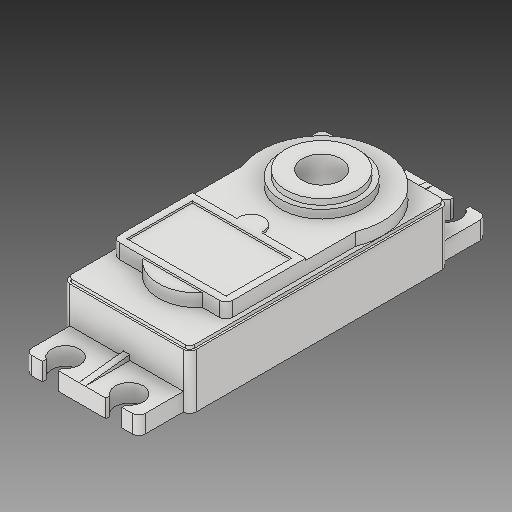
# Autodesk Inventor part: Top
Saved by Autodesk Inventor 2018 (Build 220112000, 112)
## iProperties
Created: 2016-09-26
Part Number: Top
Material: Plástico ABS
Document SubType Name: Modeling
Designer: Julian
Density: 1.06 g/cm^3
Appearance: Suave - Blanco
Author: Julian
Autodesk Inventor part; units mm, degrees
ref_plane "YZ Plane" through (0, 0, 0) normal (1, 0, 0) x (0, 1, 0)
ref_plane "XZ Plane" through (0, 0, 0) normal (0, 1, 0) x (-1, 0, 0)
ref_plane "XY Plane" through (0, 0, 0) normal (0, 0, 1) x (1, 0, 0)
sketch "Boceto1" plane through (0, 0, 0) normal (0, 1, 0) x (-1, 0, 0)
  line L0 (9.9, 20.3) -> (-9.9, 20.3)
  line L1 (-9.9, 20.3) -> (-9.9, -20.3)
  line L2 (-9.9, -20.3) -> (9.9, -20.3)
  line L3 (9.9, -20.3) -> (9.9, 20.3)
  line L4 (9.9, 20.3) -> (-9.9, -20.3) construction
  line L5 (-9.9, 20.3) -> (9.9, -20.3) construction
  point P0 (0, 0)
  dimension "d0" = 19.8
  dimension "d1" = 40.6
  constraints: 12 end point, 2 midpoint, 2 parallel, 1 horizontal, 1 perpendicular
  measures "d0" distance of L2.end L1.end
  measures "d1" distance of L1.end L0.end
extrude "Extrusión1" add sketch "Boceto1" against normal blind 9
sketch "Boceto2" plane through (0, 0, 0) normal (0, 1, 0) x (1, 0, 0)
  circle A0 centre (0, 10.3) radius 3
  line L0 (9.9, 20.3) -> (-9.9, 20.3) projected
  point P0 (0, 0)
  dimension "d4" = 6
  dimension "d5" = 10
  constraints: 1 centre point
  measures "d4" diameter of A0
  measures "d5" distance from line of L0 A0.centre
extrude "Extrusión2" cut sketch "Boceto2" against normal through all
sketch "Boceto5" plane through (0, -9, 0) normal (0, -1, 0) x (1, 0, 0)
  line L0 (-8.9, 20.3) -> (8.9, 20.3)
  line L1 (8.9, 20.3) -> (8.9, 27.3)
  line L2 (8.9, 27.3) -> (-8.9, 27.3)
  line L3 (-8.9, 27.3) -> (-8.9, 20.3)
  line L4 (-8.9, 20.3) -> (8.9, 27.3) construction
  line L5 (8.9, 20.3) -> (-8.9, 27.3) construction
  line L6 (-9.9, 27.3) -> (9.9, 27.3)
  line L7 (9.9, 20.3) -> (-9.9, 20.3) projected
  point P0 (0, 0)
  point P1 (0, 0)
  point P2 (0, 23.8)
  dimension "d23" = 17.8
  dimension "d24" = 7
  constraints: 14 end point, 2 collinear, 2 midpoint, 2 parallel, 1 horizontal, 1 perpendicular
  measures "d23" distance of L2.end L1.end
  measures "d24" distance of L1.end L0.end
extrude "Extrusión5" add sketch "Boceto5" against normal blind 2.8
sketch "Boceto6" plane through (0, -6.2, 0) normal (0, 1, 0) x (1, 0, 0)
  arc A0 (-3.75, -26.7004) -> (-6.25, -26.7004) centre (-5, -24.89) ccw
  line L0 (-8.9, -27.3) -> (8.9, -27.3)
  line L1 (-3.75, -27.3) -> (-6.25, -27.3)
  line L2 (-6.25, -27.3) -> (-6.25, -26.7)
  line L3 (-3.75, -26.7) -> (-3.75, -27.3)
  line L4 (0, -27.3) -> (0, -23.9124)
  line L5 (-8.9, -20.3) -> (-8.9, -27.3)
  line L6 (-8.9, -20.3) -> (8.9, -20.3) projected
  line L7 (-8.3229, -20.3) -> (8.9, -20.3)
  line L8 (8.9, -20.3) -> (8.9, -27.3)
  point P0 (0, 0)
  point P1 (0, 0)
  dimension "d27" = 4.4
  dimension "d28" = 2.41
  dimension "d29" = 5
  dimension "d30" = 2.65
  dimension "d31" = 0.6
  constraints: 16 end point, 3 point on line, 2 horizontal, 2 parallel, 2 perpendicular, 2 point on circle, 2 vertical, 1 centre point, 1 midpoint
  measures "d27" diameter of A0
  measures "d28" distance from line of L0 A0.centre
  measures "d29" distance from line of L4 A0.centre
  measures "d30" distance between parallel lines of L5 L2
  measures "d31" distance of L3.start L1.start
extrude "Extrusión6" cut sketch "Boceto6" against normal through all contours L3 L0 L2 A0
sketch "Boceto8" plane through (0, 0, 0) normal (1, 0, 0) x (0, 1, 0)
  line L0 (-6.2, 27.3) -> (-5.4, 20.3)
  line L1 (-5.4, 20.3) -> (-6.2, 20.3)
  line L2 (-6.2, 20.3) -> (-6.2, 27.3)
  point P0 (0, 0)
  dimension "d34" = 0.8
  constraints: 6 end point, 1 horizontal, 1 perpendicular
  measures "d34" distance of L1.end L0.end
extrude "Extrusión7" add sketch "Boceto8" along normal mid plane 1
mirror "Simetría3" about plane through (0, 0, 0) normal (1, 0, 0) of "Extrusión6"
mirror "Simetría4" about plane through (0, 0, 0) normal (0, 0, 1) of "Extrusión5", "Extrusión6", "Simetría3", "Extrusión7"
sketch "Boceto9" plane through (0, 0, 0) normal (0, 1, 0) x (1, 0, 0)
  circle A0 centre (0, 10.3) radius 3 projected
  line L0 (-8.9, -13.5986) -> (8.9, -13.5986)
  line L1 (8.9, -13.5986) -> (8.9, 6.7014)
  line L2 (-8.9, 6.7014) -> (-8.9, -13.5986)
  line L3 (-8.9, -13.5986) -> (5.885, 8.9919) construction
  line L4 (8.9, -13.5986) -> (-5.885, 8.9919) construction
  arc A1 (8.9, 6.7014) -> (-8.9, 6.7014) centre (0, 10.3) ccw
  line L5 (9.9, 20.3) -> (-9.9, 20.3) projected
  point P0 (0, 0)
  dimension "d40" = 9.6
  dimension "d42" = 20.3
  dimension "d61" = 17.8
  constraints: 10 end point, 2 parallel, 2 point on circle, 2 point on line, 1 centre point, 1 horizontal, 1 perpendicular
  measures "d40" radius of A1
  measures "d42" distance of L0.end L1.end
  measures "d61" distance between parallel lines of L1 L2
extrude "Extrusión8" add sketch "Boceto9" along normal blind 2
sketch "Boceto11" plane through (0, 2, 0) normal (0, 1, 0) x (1, 0, 0)
  line L0 (-8.9, -13.5986) -> (8.9, -13.5986) projected
  line L1 (5.2244, -15.7986) -> (5.2244, -13.5986)
  arc A0 (-4.1756, -13.5986) -> (5.2244, -13.5986) centre (0.5244, -9.6782) ccw
  line L2 (-4.1756, -13.5986) -> (5.2244, -13.5986)
  point P0 (0, 0)
  dimension "d50" = 2.2
  dimension "d51" = 9.4
  constraints: 4 end point, 2 point on circle, 1 centre point, 1 collinear, 1 point on line
  measures "d50" distance edge to line of A0 L0
  measures "d51" distance of L1.end L2.start
extrude "Extrusión9" add sketch "Boceto11" against normal blind 2
sketch "Boceto12" plane through (0, 2, 0) normal (0, 1, 0) x (1, 0, 0)
  circle A0 centre (0, 10.3) radius 6.4
  circle A1 centre (0, 10.3) radius 3 projected
  point P0 (0, 0)
  dimension "d54" = 12.8
  constraints: 1 centre point, 1 coincident
  measures "d54" diameter of A0
extrude "Extrusión10" add sketch "Boceto12" along normal blind 1.3
sketch "Boceto13" plane through (0, 3.3, -10.3) normal (0, 1, 0) x (1, 0, 0)
  circle A0 centre (0, 0) radius 5.6
  circle A1 centre (0, 0) radius 3 projected
  point P0 (0, -10.3)
  dimension "d57" = 11.2
  constraints: 1 centre point
  measures "d57" diameter of A0
extrude "Extrusión11" add sketch "Boceto13" along normal blind 0.9
sketch "Boceto15" plane through (0, 2, 0) normal (0, 1, 0) x (1, 0, 0)
  line L0 (8.9, 6.7014) -> (8.9, -13.5986) projected
  line L1 (-8.9, -13.5986) -> (8.9, -13.5986)
  line L2 (8.9, -13.5986) -> (8.9, -1.0986)
  line L3 (8.9, -1.0986) -> (-8.9, -1.0986)
  line L4 (-8.9, -1.0986) -> (-8.9, -13.5986)
  line L5 (-8.9, -13.5986) -> (8.9, -1.0986) construction
  line L6 (8.9, -13.5986) -> (-8.9, -1.0986) construction
  line L7 (-8.9, -13.5986) -> (-4.1756, -13.5986) projected
  line L8 (-7.8, -12.4986) -> (7.8, -12.4986)
  line L9 (7.8, -12.4986) -> (7.8, -2.1986)
  line L10 (7.8, -2.1986) -> (-7.8, -2.1986)
  line L11 (-7.8, -2.1986) -> (-7.8, -12.4986)
  point P0 (0, 0)
  point P1 (0, -7.3486)
  dimension "d62" = 12.5
  dimension "d63" = 1.1
  constraints: 20 end point, 4 parallel, 2 midpoint, 2 perpendicular, 1 collinear, 1 horizontal, 1 point on line, 3 other
  measures "d62" distance of L2.end L1.end
  measures "d63" distance between parallel lines of L4 L11
extrude "Extrusión12" add sketch "Boceto15" along normal blind 0.3
sketch "Boceto16" plane through (0, 2.3, 0) normal (0, 1, 0) x (1, 0, 0)
  arc A0 (1.91, -1.0986) -> (-1.91, -1.0986) centre (0, -0.7586) ccw
  line L0 (-7.8, -2.1986) -> (7.8, -2.1986) projected
  line L1 (8.9, -1.0986) -> (-8.9, -1.0986) projected
  point P0 (0, 0)
  dimension "d66" = 3.88
  dimension "d67" = 1.44
  constraints: 2 point on circle, 2 point on line, 1 centre point
  measures "d66" diameter of A0
  measures "d67" distance from line of L0 A0.centre
extrude "Extrusión13" add sketch "Boceto16" against normal blind 0.3
sketch "Boceto17" plane through (0, 0, 0) normal (0, 1, 0) x (1, 0, 0)
  line L0 (-9.9, 20.3) -> (-9.9, -20.3) projected
  line L1 (9.9, -20.3) -> (9.9, 20.3) projected
  line L2 (-9.9, -20.3) -> (9.9, -20.3) projected
  line L3 (9.9, 20.3) -> (-9.9, 20.3) projected
  line L4 (-9.6, -20) -> (-9.6, 20)
  line L5 (-9.6, 20) -> (9.6, 20)
  line L6 (9.6, 20) -> (9.6, -20)
  line L7 (9.6, -20) -> (-9.6, -20)
  point P0 (0, 0)
  dimension "d70" = 0.3
  constraints: 8 end point, 3 other
  measures "d70" distance between parallel lines of L0 L4
extrude "Extrusión14" cut sketch "Boceto17" against normal blind 0.5
fillet "Empalme1" radius 1 10 edges at (9.9, -4.75, 20.3) (8.9, -7.6, 27.3) (-8.9, -7.6, 27.3) (-9.9, -4.75, 20.3) (8.9, 1.15, 13.5986) (-8.9, 1.15, 13.5986) (9.9, -4.75, -20.3) (-9.9, -4.75, -20.3) (-8.9, -7.6, -27.3) (8.9, -7.6, -27.3)
fillet "Empalme2" radius 0.7 4 edges at (9.6, -0.25, 20) (-9.6, -0.25, 20) (9.6, -0.25, -20) (-9.6, -0.25, -20)
sketch "Boceto18" plane through (0, 2, 0) normal (0, 1, 0) x (1, 0, 0)
  point P0 (0, 0)
